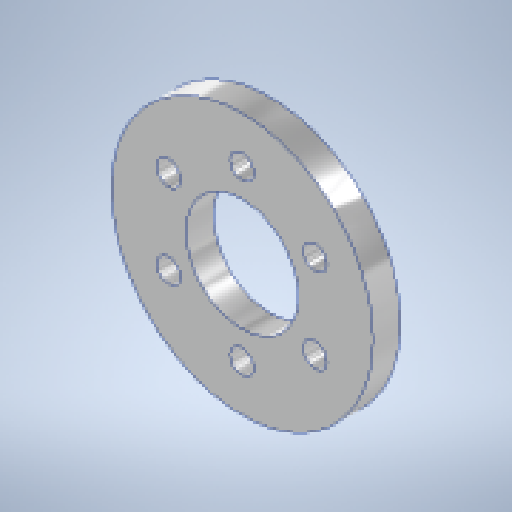
# Autodesk Inventor part: servoplate_forR3
Saved by Autodesk Inventor 2024.3 (Build 283343010, 343A)
## iProperties
Created: 2025-05-25
Part Number: servoplate_forR3
Material: アルミニウム 6061
Document SubType Name: Modeling
Designer: kshau
Density: 2.7 g/cm^3
Appearance: アルミニウム - フラット
Author: kshau
Autodesk Inventor part; units mm, degrees
ref_plane "YZ Plane" through (0, 0, 0) normal (1, 0, 0) x (0, 1, 0)
ref_plane "XZ Plane" through (0, 0, 0) normal (0, 1, 0) x (-1, 0, 0)
ref_plane "XY Plane" through (0, 0, 0) normal (0, 0, 1) x (1, 0, 0)
sketch "スケッチ1" plane through (0, 0, 0) normal (0, 0, 1) x (1, 0, 0)
  circle A0 centre (0, 0) radius 23.5
  dimension "d0" = 47
  constraints: 1 centre point, 1 coincident
  measures "d0" diameter of A0
extrude "押し出し1" add sketch "スケッチ1" along normal blind 5
sketch "スケッチ2" plane through (0, 0, 5) normal (0, 0, 1) x (1, 0, 0)
  circle A0 centre (0, 0) radius 15.18
  point P0 (0, 15.18)
  point P1 (-13.1463, 7.59)
  point P2 (-13.1463, -7.59)
  point P3 (0, -15.18)
  point P4 (13.1463, -7.59)
  point P5 (13.1463, 7.59)
  dimension "d3" = 30.36
  dimension "d6" = 360
  constraints: 1 coincident, 1 vertical alignment, 9 other
hole "穴1" at (0, 15.18, 5) at (-13.1463, 7.59, 5) at (-13.1463, -7.59, 5) at (0, -15.18, 5) at (13.1463, -7.59, 5) at (13.1463, 7.59, 5) direction (0, 0, -1) diameter 4.3 end through all
sketch "スケッチ3" plane through (0, 0, 5) normal (0, 0, 1) x (1, 0, 0)
  circle A0 centre (0, 0) radius 10.1
  dimension "d15" = 20.2
  constraints: 1 centre point, 1 coincident
  measures "d15" diameter of A0
extrude "押し出し2" cut sketch "スケッチ3" against normal blind 5
